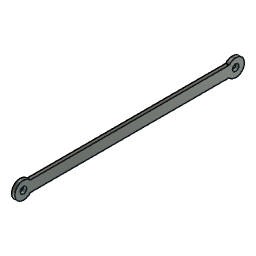
palochicov2 v2 (Autodesk Fusion 360 design; units mm, degrees)
Autodesk Fusion 360 part; units mm, degrees
sketch "Boceto1" plane through (0, 0, 0) normal (1, 0, 0) x (0, 1, 0)
  line L0 (0, 0) -> (90, 0)
  line L1 (90, 5) -> (0, 5)
  line L2 (0, 5) -> (-0.8775, 5)
  line L3 (90, 5) -> (90.8775, 5)
  line L4 (0, 0) -> (-2, 0)
  line L5 (90, 0) -> (91.5, 0)
  circle A0 centre (94, 2.5) radius 1.5
  circle A1 centre (-4, 2.5) radius 1.5
  arc A2 (-0.8775, 5) -> (-0.8775, 0) centre (-4, 2.5) ccw
  arc A3 (90.8775, 0) -> (90.8775, 5) centre (94, 2.5) ccw
  dimension "d1" = 90
  dimension "d2" = 5
  dimension "d4" = 3
  dimension "d5" = 3
  constraint horizontal L0
  constraint horizontal L1
  constraint coincident L0.start L4.start
  constraint horizontal L4
  constraint concentric A0 A3
  constraint concentric A1 A2
  constraint coincident L4 A2.end
  constraint coincident L5 A3.start
  measures "d1" distance of L0.start L0.end
  measures "d2" distance of L0.start L1.end
  measures "d4" diameter of A0
  measures "d5" diameter of A1
extrude "Extruir1" add sketch "Boceto1" along normal blind 1.5
sketch "Boceto2" plane through (1.5, 0, 0) normal (1, 0, 0) x (0, 1, 0)
  circle A0 centre (94, 2.5) radius 1.5
  circle A1 centre (-4, 2.5) radius 1.5
  line L0 (-0.8775, 0) -> (90.8775, 0)
  arc A2 (90.8775, 0) -> (90.8775, 5) centre (94, 2.5) ccw
  line L1 (90.8775, 5) -> (-0.8775, 5)
  arc A3 (-0.8775, 5) -> (-0.8775, 0) centre (-4, 2.5) ccw
